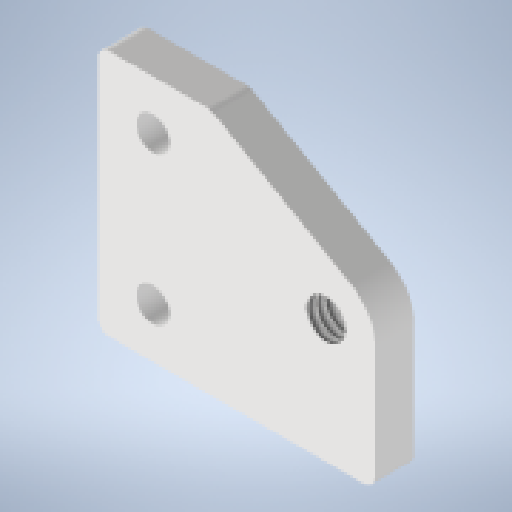
# Autodesk Inventor part: Gas Strut Lower Plate
Saved by Autodesk Inventor 2024 (Build 280153000, 153)
## iProperties
Created: 2024-11-25
Part Number: Gas Strut Lower Plate
Material: Generic
Document SubType Name: Modeling
Designer: Ishaan
Density: 1 g/cm^3
Appearance: Default
Author: Ishaan
Autodesk Inventor part; units mm, degrees
ref_plane "YZ Plane" through (0, 0, 0) normal (1, 0, 0) x (0, 1, 0)
ref_plane "XZ Plane" through (0, 0, 0) normal (0, 1, 0) x (-1, 0, 0)
ref_plane "XY Plane" through (0, 0, 0) normal (0, 0, 1) x (1, 0, 0)
sketch "Sketch1" plane through (0, 0, 0) normal (0, 0, 1) x (1, 0, 0)
  line L0 (22.5, -20) -> (-22.5, -20)
  line L1 (-22.5, -20) -> (-22.5, 20)
  line L2 (-22.5, 20) -> (22.5, 20)
  line L3 (22.5, 20) -> (22.5, -20)
  line L4 (22.5, -20) -> (-22.5, 20) construction
  line L5 (-22.5, -20) -> (22.5, 20) construction
  circle A0 centre (14.5, 0) radius 8
  line L6 (18.5, 6.9282) -> (-4.141, 20)
  circle A1 centre (-13.5, 12) radius 2.7
  circle A2 centre (-13.5, -12) radius 2.7
  point P0 (0, 0)
  point P1 (22.5, 0)
  dimension "d4" = 16
  dimension "d0" = 40
  dimension "d1" = 9
  dimension "d2" = 8
  dimension "d3" = 8
  dimension "d5" = 28
  dimension "d6" = 30
  dimension "d7" = 20
  dimension "d8" = 5.4
  constraints: 14 end point, 3 coincident, 2 centre point, 2 midpoint, 2 parallel, 1 equal radius, 1 horizontal, 1 perpendicular, 1 point on line, 1 vertical, 1 vertical alignment, 4 other
  measures "d0" distance of L0.end L1.end
  measures "d1" distance from line of L1 point (-13.5, 12)
  measures "d2" distance from line of L2 point (-13.5, 12)
  measures "d3" distance from line of L0 point (-13.5, -12)
  measures "d5" horizontal distance of point (14.5, 0) point (-13.5, 12)
  measures "d6" angle of L2 L6
  measures "d7" distance from line of L0 point (14.5, 0)
  measures "d8" diameter of A1
extrude "Extrusion1" add sketch "Sketch1" along normal blind 6.35 contours L0 L1 L2 L6 A0 L3 | A0
sketch "Sketch2" plane through (0, 0, 6.35) normal (0, 0, 1) x (1, 0, 0)
  arc A0 (22.5, 0) -> (18.5, 6.9282) centre (14.5, 0) ccw projected
  point P0 (0, 0)
  constraints: 1 coincident
hole "Hole1" at (14.5, 0, 6.35) direction (0, 0, -1) diameter 6.4008 end through all thread size "5/16-18 UNC" class "2B" standard "ANSI Unified Screw Threads"
fillet "Fillet1" radius 2 4 edges at (-22.5, 20, 3.175) (-22.5, -20, 3.175) (22.5, -20, 3.175) (-4.141, 20, 3.175)
equation "\"d3\" = d2"
body "Solid1"
